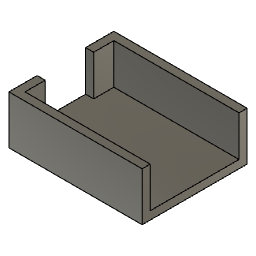
luos usg gate holder v1 (Autodesk Fusion 360 design; units mm, degrees)
Autodesk Fusion 360 part; units mm, degrees
note: some values were not read from the file. Set by a fixed rule: which face or edge a step refers to.
sketch "Sketch1" plane through (0, 0, 0) normal (0, 0, 1) x (1, 0, 0)
  line L0 (0, 0) -> (31, 0)
  line L1 (31, 0) -> (31, 26)
  line L2 (31, 26) -> (0, 26)
  line L3 (0, 26) -> (0, 0)
  dimension "d1" = 31
  dimension "d2" = 26
  constraint horizontal L0
  constraint vertical L1
  constraint horizontal L2
  constraint vertical L3
  constraint coincident L0.start L3.end
  measures "d1" distance of L0.start L0.end
  measures "d2" distance of L0.start L2.end
extrude "Extrude1" add sketch "Sketch1" along normal blind 10 contours L0 L1 L2 L3 picked at (10.333333, 17.333333)
shell "Shell1" thickness 2 removed faces 1 at (10.333333, 17.333333, 10)
extrude "Extrude2" cut 1 faces at (2, 16.666667, 4.666667) along direction (-1, 0, 0) blind 10
extrude "Extrude3" cut 1 faces at (29, 16.666667, 7.333333) along direction (1, 0, 0) blind 20
sketch "Sketch2" plane through (0, 26, 0) normal (0, 1, 0) x (-1, 0, 0)
  line L0 (-31, 0) -> (0, 0)
  line L1 (0, 0) -> (0, 10)
  line L2 (0, 10) -> (-31, 10)
  line L3 (-31, 10) -> (-31, 0)
  line L4 (0, 0) -> (2, 0)
  line L5 (2, 0) -> (2, 10.022047)
  line L6 (2, 10.022047) -> (0, 10.022047)
  line L7 (0, 10.022047) -> (0, 0)
  dimension "d10" = 2
  constraint horizontal L4
  constraint vertical L5
  constraint horizontal L6
  constraint vertical L7
  constraint coincident L0.end L1.start
  measures "d10" distance of L0.end L4.end
extrude "Extrude4" add sketch "Sketch2" against normal blind 7 contours L1 L4 L5 L6 L7 picked at (1.333333, 6.674016)
sketch "Sketch3" plane through (0, 0, 0) normal (0, 1, 0) x (1, 0, 0)
  line L0 (0, 0) -> (-2, 0)
  line L1 (-2, 0) -> (-2, -10)
  line L2 (-2, -10) -> (0, -10)
  line L3 (0, -10) -> (0, 0)
  dimension "d13" = 2
  constraint horizontal L0
  constraint vertical L1
  constraint horizontal L2
  constraint vertical L3
  constraint coincident L0.start L3.end
  measures "d13" distance of L0.start L0.end
extrude "Extrude5" add sketch "Sketch3" along normal blind 7 contours L0 L1 L2 L3 picked at (-1.333333, -3.333333)
extrude "Extrude6" cut 1 faces at (-1.333333, 23.666667, 10.022047) along direction (0, 0, -1) blind 0.022
extrude "Extrude7" cut 1 faces at (-1.333333, 23.666667, 10.000047) along direction (0, 0, -1) blind 0.000048
extrude "Extrude8" add 1 faces at (0, 15, 0.666667) along direction (-1, 0, 0) blind 2
extrude "Extrude9" add 2 faces at (-1.333333, 3, 10) (10.333333, 0.666667, 10) along direction (0, 0, 1) blind 2
extrude "Extrude10" add 2 faces at (-1.333333, 23, 9.999999) (10.333333, 25.333333, 10) along direction (0, 0, 1) blind 2
equation "d18 = -4.768E-05 mm"
